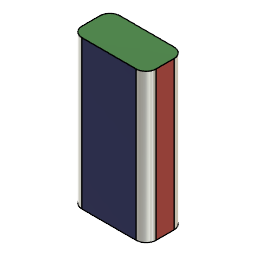
Raven Electronics Assembly (Autodesk Fusion 360 archive; units mm, degrees)
design "2s3000Mah Copy"
Autodesk Fusion 360 part; units mm, degrees
sketch "Sketch1" plane through (0, 0, 0) normal (0, 0, 1) x (1, 0, 0)
  line L0 (18.5, 9.5) -> (-18.5, 9.5)
  line L1 (-18.5, 9.5) -> (-18.5, -9.5)
  line L2 (-18.5, -9.5) -> (18.5, -9.5)
  line L3 (18.5, -9.5) -> (18.5, 9.5)
  line L4 (18.5, 9.5) -> (-18.5, -9.5) construction
  line L5 (-18.5, 9.5) -> (18.5, -9.5) construction
  dimension "d3" = 19
  dimension "d4" = 37
  constraint horizontal L0
  constraint perpendicular L0 L1
  constraint parallel L0 L2
  constraint parallel L1 L3
  constraint coincident L4 origin
  constraint coincident L5 origin
  measures "d3" distance of L0.end L1.end
  measures "d4" distance of L0.start L0.end
extrude "Extrude1" add sketch "Sketch1" along normal blind 74
fillet "Fillet1" radius 5 4 edges at (-18.5, -9.5, 37) (18.5, 9.5, 37) (18.5, -9.5, 37) (-18.5, 9.5, 37)

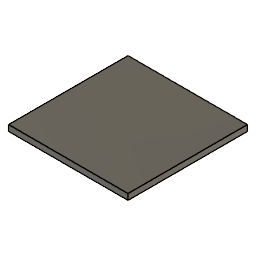
design "Electronics Case Top"
Autodesk Fusion 360 part; units mm, degrees
sketch "Sketch1" plane through (0, 0, 0) normal (0, 0, 1) x (1, 0, 0)
  line L0 (0, 0) -> (60, 0)
  line L1 (60, 0) -> (60, 60)
  line L2 (60, 60) -> (0, 60)
  line L3 (0, 60) -> (0, 0)
  dimension "d1" = 60
  dimension "d2" = 60
  constraint horizontal L0
  constraint vertical L1
  constraint horizontal L2
  constraint vertical L3
  constraint coincident L0.start L3.end
  measures "d1" distance of L0.start L0.end
  measures "d2" distance of L0.start L2.end
extrude "Extrude1" add sketch "Sketch1" along normal blind 3

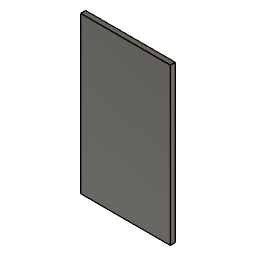
design "Electronics Case Right Wall"
Autodesk Fusion 360 part; units mm, degrees
sketch "Sketch1" plane through (0, 0, 0) normal (0, 1, 0) x (1, 0, 0)
  line L0 (0, 0) -> (54, 0)
  line L1 (54, 0) -> (54, -94)
  line L2 (54, -94) -> (0, -94)
  line L3 (0, -94) -> (0, 0)
  dimension "d1" = 54
  dimension "d2" = 94
  constraint horizontal L0
  constraint vertical L1
  constraint horizontal L2
  constraint vertical L3
  constraint coincident L0.start L3.end
  measures "d1" distance of L0.start L0.end
  measures "d2" distance of L0.start L2.end
extrude "Extrude1" add sketch "Sketch1" along normal blind 3

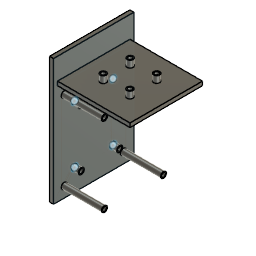
design "Electronics Case Back wall"
Autodesk Fusion 360 part; units mm, degrees
sketch "Sketch1" plane through (0, 0, 0) normal (1, 0, 0) x (0, 1, 0)
  line L0 (0, 0) -> (60, 0)
  line L1 (60, 0) -> (60, 94)
  line L2 (60, 94) -> (0, 94)
  line L3 (0, 94) -> (0, 0)
  dimension "d1" = 60
  dimension "d2" = 94
  constraint horizontal L0
  constraint vertical L1
  constraint horizontal L2
  constraint vertical L3
  constraint coincident L0.start L3.end
  measures "d1" distance of L0.start L0.end
  measures "d2" distance of L0.start L2.end
extrude "Extrude1" add sketch "Sketch1" along normal blind 3
sketch "Sketch2" plane through (3, 0, 0) normal (1, 0, 0) x (0, 1, 0)
  line L0 (0, 94) -> (0, 0)
  line L1 (0, 0) -> (60, 0)
  line L2 (60, 0) -> (60, 94)
  line L3 (60, 94) -> (0, 94)
  line L4 (0, 0) -> (0, 75)
  line L5 (0, 75) -> (60, 75)
  line L6 (60, 75) -> (60, 78)
  line L7 (60, 78) -> (0, 78)
  line L8 (0, 78) -> (0, 75)
  dimension "d5" = 75
  dimension "d6" = 60
  dimension "d7" = 3
  constraint coincident L0.end L1.start
  constraint perpendicular L1 L4
  constraint horizontal L5
  constraint vertical L6
  constraint horizontal L7
  constraint vertical L8
  measures "d5" distance of L0.end L4.end
  measures "d6" distance of L4.end L5.end
  measures "d7" distance of L4.end L7.end
extrude "Extrude2" add sketch "Sketch2" along normal blind 54 contours L0 L2 L5 L6 L7 L8
sketch "Sketch3" plane through (0, 0, 0) normal (0, -1, 0) x (1, 0, 0)
  line L0 (0, 94) -> (0, 0)
  line L1 (0, 0) -> (3, 0)
  line L2 (3, 0) -> (3, 75)
  line L3 (3, 75) -> (57, 75)
  line L4 (57, 75) -> (57, 78)
  line L5 (57, 78) -> (3, 78)
  line L6 (3, 78) -> (3, 94)
  line L7 (3, 94) -> (0, 94)
  line L8 (3, 75) -> (57, 75)
  line L9 (57, 75) -> (57, 78)
  line L10 (57, 78) -> (3, 78)
  line L11 (3, 78) -> (3, 75)
  constraint horizontal L8
  constraint vertical L9
  constraint horizontal L10
  constraint vertical L11
  constraint coincident L4.end L5.start
  constraint coincident L2.end L3.start
extrude "Extrude3" cut sketch "Sketch3" against normal blind 3 contours L3 L4 L5 L8 L9 L10 L11
sketch "Sketch4" plane through (0, 60, 0) normal (0, 1, 0) x (-1, 0, 0)
  line L0 (0, 0) -> (0, 94)
  line L1 (0, 94) -> (-3, 94)
  line L2 (-3, 94) -> (-3, 78)
  line L3 (-3, 78) -> (-57, 78)
  line L4 (-57, 78) -> (-57, 75)
  line L5 (-57, 75) -> (-3, 75)
  line L6 (-3, 75) -> (-3, 0)
  line L7 (-3, 0) -> (0, 0)
  line L8 (-57, 75) -> (-3, 75)
  line L9 (-3, 75) -> (-3, 78)
  line L10 (-3, 78) -> (-57, 78)
  line L11 (-57, 78) -> (-57, 75)
  constraint horizontal L8
  constraint vertical L9
  constraint horizontal L10
  constraint vertical L11
  constraint coincident L2.end L3.start
  constraint coincident L4.end L5.start
extrude "Extrude4" cut sketch "Sketch4" against normal blind 3 contours L3 L4 L5 L8 L9 L10 L11
sketch "Sketch5" plane through (3, 0, 0) normal (1, 0, 0) x (0, 1, 0)
  line L0 (57, 75) -> (3, 75)
  line L1 (3, 75) -> (3, 78)
  line L2 (3, 78) -> (57, 78)
  line L3 (57, 78) -> (57, 75)
  line L4 (60, 0) -> (60, 94)
  line L5 (60, 94) -> (0, 94)
  line L6 (0, 94) -> (0, 0)
  line L7 (0, 0) -> (60, 0)
sketch "Sketch6" plane through (3, 0, 0) normal (1, 0, 0) x (0, 1, 0)
  circle A0 centre (44.31, 16.105) radius 1.5
  circle A1 centre (44.31, 16.105) radius 2.25
  circle A2 centre (15.69, 16.105) radius 1.5
  circle A3 centre (15.69, 16.105) radius 2.25
  circle A4 centre (15.69, 58.895) radius 1.5
  circle A5 centre (15.69, 58.895) radius 2.25
  circle A6 centre (44.31, 58.895) radius 1.5
  circle A7 centre (44.31, 58.895) radius 2.25
  dimension "d25" = 3
  dimension "d26" = 4.5
  dimension "d27" = 28.62
  dimension "d28" = 3
  dimension "d29" = 4.5
  dimension "d30" = 42.79
  dimension "d31" = 3
  dimension "d32" = 4.5
  dimension "d33" = 42.79
  dimension "d34" = 3
  dimension "d35" = 4.5
  constraint concentric A0 A1
  constraint concentric A2 A3
  constraint concentric A4 A5
  constraint concentric A6 A7
  measures "d25" diameter of A0
  measures "d26" diameter of A1
  measures "d27" distance of A0.centre A2.centre
  measures "d28" diameter of A2
  measures "d29" diameter of A3
  measures "d30" distance of A2.centre A4.centre
  measures "d31" diameter of A4
  measures "d32" diameter of A5
  measures "d33" distance of A0.centre A6.centre
  measures "d34" diameter of A6
  measures "d35" diameter of A7
extrude "Extrude6" add sketch "Sketch6" along normal blind 5
sketch "Sketch7" plane through (0, 0, 78) normal (0, 0, 1) x (-1, 0, 0)
  line L0 (-57, -57) -> (-3, -57)
  line L1 (-3, -57) -> (-3, -3)
  line L2 (-3, -3) -> (-57, -3)
  line L3 (-57, -3) -> (-57, -57)
  line L4 (-57, -3) -> (-57, -20)
  line L5 (-57, -20) -> (-39.9, -20)
  circle A0 centre (-39.9, -20) radius 1.5
  circle A1 centre (-39.9, -20) radius 2.25
  line L6 (-39.9, -20) -> (-20.1, -20)
  circle A2 centre (-20.1, -20) radius 1.5
  circle A3 centre (-20.1, -20) radius 2.25
  line L7 (-20.1, -20) -> (-20.1, -40)
  circle A4 centre (-20.1, -40) radius 1.5
  circle A5 centre (-20.1, -40) radius 2.25
  line L8 (-39.9, -20) -> (-39.9, -40)
  circle A6 centre (-39.9, -40) radius 1.5
  circle A7 centre (-39.9, -40) radius 2.25
  dimension "d38" = 17
  dimension "d39" = 17.1
  dimension "d40" = 3
  dimension "d41" = 4.5
  dimension "d42" = 19.8
  dimension "d43" = 3
  dimension "d44" = 4.5
  dimension "d45" = 20
  dimension "d46" = 3
  dimension "d47" = 4.5
  dimension "d48" = 20
  dimension "d49" = 3
  dimension "d50" = 4.5
  constraint coincident L2.end L3.start
  constraint perpendicular L2 L4
  constraint perpendicular L4 L5
  constraint coincident L5.end A0.centre
  constraint concentric A0 A1
  constraint parallel L5 L6
  constraint coincident L6.end A2.centre
  constraint concentric A2 A3
  constraint perpendicular L6 L7
  constraint coincident L7.end A4.centre
  constraint concentric A4 A5
  constraint perpendicular L6 L8
  constraint coincident L8.end A6.centre
  constraint concentric A6 A7
  measures "d38" distance of L2.end L4.end
  measures "d39" distance of L4.end L5.end
  measures "d40" diameter of A0
  measures "d41" diameter of A1
  measures "d42" distance of L5.end L6.end
  measures "d43" diameter of A2
  measures "d44" diameter of A3
  measures "d45" distance of L6.end L7.end
  measures "d46" diameter of A4
  measures "d47" diameter of A5
  measures "d48" distance of L5.end L8.end
  measures "d49" diameter of A6
  measures "d50" diameter of A7
extrude "Extrude7" add sketch "Sketch7" along normal blind 5 contours L5 A0 A1 L6 | L5 A0 A1 L8 | A0 A1 L6 L8 | L6 A2 A3 L7 | L6 A2 A3 L7 | A5 | A7
sketch "Sketch8" plane through (3, 0, 0) normal (1, 0, 0) x (0, 1, 0)
  line L0 (0, 0) -> (8, 0)
  line L1 (8, 0) -> (8, 8)
  circle A0 centre (8, 8) radius 1.5
  circle A1 centre (8, 8) radius 2.25
  line L2 (60, 0) -> (52, 0)
  line L3 (52, 0) -> (52, 8)
  line L4 (52, 8) -> (60, 8)
  line L5 (60, 8) -> (60, 0)
  circle A2 centre (52, 8) radius 1.5
  circle A3 centre (52, 8) radius 2.25
  line L6 (60, 75) -> (52, 75)
  line L7 (52, 75) -> (52, 67)
  line L8 (52, 67) -> (60, 67)
  line L9 (60, 67) -> (60, 75)
  circle A4 centre (52, 67) radius 1.5
  circle A5 centre (52, 67) radius 2.25
  line L10 (0, 75) -> (8, 75)
  line L11 (8, 75) -> (8, 67)
  line L12 (8, 67) -> (0, 67)
  line L13 (0, 67) -> (0, 75)
  circle A6 centre (8, 67) radius 1.5
  circle A7 centre (8, 67) radius 2.25
  dimension "d53" = 8
  dimension "d54" = 8
  dimension "d55" = 3
  dimension "d56" = 4.5
  dimension "d57" = 8
  dimension "d58" = 8
  dimension "d59" = 3
  dimension "d60" = 4.5
  dimension "d61" = 8
  dimension "d62" = 8
  dimension "d63" = 3
  dimension "d64" = 4.5
  dimension "d65" = 8
  dimension "d66" = 8
  dimension "d67" = 3
  dimension "d68" = 4.5
  constraint coincident L0.start origin
  constraint horizontal L0
  constraint perpendicular L0 L1
  constraint coincident L1.end A0.centre
  constraint concentric A0 A1
  constraint horizontal L2
  constraint vertical L3
  constraint horizontal L4
  constraint vertical L5
  constraint coincident L3.end L4.start
  constraint concentric A2 A3
  constraint horizontal L6
  constraint vertical L7
  constraint horizontal L8
  constraint vertical L9
  constraint coincident L7.end L8.start
  constraint concentric A4 A5
  constraint horizontal L10
  constraint vertical L11
  constraint horizontal L12
  constraint vertical L13
  constraint coincident L11.end L12.start
  constraint concentric A6 A7
  measures "d53" distance of L0.start L0.end
  measures "d54" distance of L0.end L1.end
  measures "d55" diameter of A0
  measures "d56" diameter of A1
  measures "d57" distance of L2.start L2.end
  measures "d58" distance of L2.start L4.end
  measures "d59" diameter of A2
  measures "d60" diameter of A3
  measures "d61" distance of L6.start L6.end
  measures "d62" distance of L6.start L8.end
  measures "d63" diameter of A4
  measures "d64" diameter of A5
  measures "d65" distance of L10.start L10.end
  measures "d66" distance of L10.start L12.end
  measures "d67" diameter of A6
  measures "d68" diameter of A7
extrude "Extrude8" add sketch "Sketch8" along normal blind 30 contours A1 | L3 L4 A2 A3 | L3 L4 A2 A3 | L7 L8 A4 A5 | L7 L8 A4 A5 | L11 L12 A6 A7 | L11 L12 A6 A7

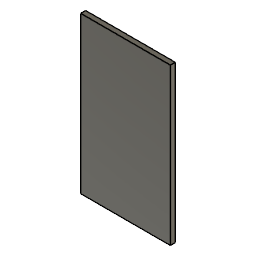
design "Electronics Case Left wall"
Autodesk Fusion 360 part; units mm, degrees
sketch "Sketch1" plane through (0, 0, 0) normal (0, 1, 0) x (1, 0, 0)
  line L0 (0, 0) -> (54, 0)
  line L1 (54, 0) -> (54, -94)
  line L2 (54, -94) -> (0, -94)
  line L3 (0, -94) -> (0, 0)
  dimension "d1" = 54
  dimension "d2" = 94
  constraint horizontal L0
  constraint vertical L1
  constraint horizontal L2
  constraint vertical L3
  constraint coincident L0.start L3.end
  measures "d1" distance of L0.start L0.end
  measures "d2" distance of L0.start L2.end
extrude "Extrude1" add sketch "Sketch1" along normal blind 3

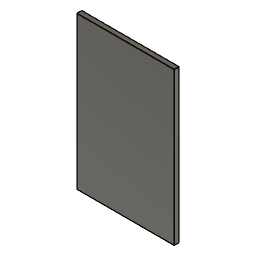
design "Electronics Case Front Wall"
Autodesk Fusion 360 part; units mm, degrees
sketch "Sketch1" plane through (0, 0, 0) normal (0, 1, 0) x (1, 0, 0)
  line L0 (0, 0) -> (60, 0)
  line L1 (60, 0) -> (60, -94)
  line L2 (60, -94) -> (0, -94)
  line L3 (0, -94) -> (0, 0)
  dimension "d1" = 60
  dimension "d2" = 94
  constraint horizontal L0
  constraint vertical L1
  constraint horizontal L2
  constraint vertical L3
  constraint coincident L0.start L3.end
  measures "d1" distance of L0.start L0.end
  measures "d2" distance of L0.start L2.end
extrude "Extrude1" add sketch "Sketch1" along normal blind 3

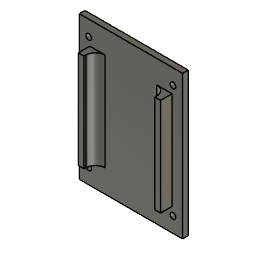
design "Electronics case internal battery shelf"
Autodesk Fusion 360 part; units mm, degrees
sketch "Sketch1" plane through (0, 0, 0) normal (0, 1, 0) x (1, 0, 0)
  line L0 (0, 0) -> (54, 0)
  line L1 (54, 0) -> (54, -75)
  line L2 (54, -75) -> (0, -75)
  line L3 (0, -75) -> (0, 0)
  dimension "d1" = 54
  dimension "d2" = 75
  constraint horizontal L0
  constraint vertical L1
  constraint horizontal L2
  constraint vertical L3
  constraint coincident L0.start L3.end
  measures "d1" distance of L0.start L0.end
  measures "d2" distance of L0.start L2.end
extrude "Extrude1" add sketch "Sketch1" along normal blind 3
sketch "Sketch2" plane through (0, 0, 0) normal (0, -1, 0) x (1, 0, 0)
  line L0 (54, 75) -> (0, 75)
  line L1 (0, 75) -> (0, 0)
  line L2 (0, 0) -> (54, 0)
  line L3 (54, 0) -> (54, 75)
  line L4 (54, 75) -> (49, 75)
  line L5 (54, 67) -> (54, 75)
  circle A0 centre (49, 67) radius 1.5
  line L6 (0, 75) -> (5, 75)
  line L7 (0, 67) -> (0, 75)
  circle A1 centre (5, 67) radius 1.5
  line L8 (0, 0) -> (5, 0)
  line L9 (0, 8) -> (0, 0)
  circle A2 centre (5, 8) radius 1.5
  line L10 (54, 0) -> (49, 0)
  line L11 (54, 8) -> (54, 0)
  circle A3 centre (49, 8) radius 1.5
  dimension "d5" = 5
  dimension "d6" = 8
  dimension "d7" = 3
  dimension "d8" = 5
  dimension "d9" = 8
  dimension "d10" = 3
  dimension "d11" = 5
  dimension "d12" = 8
  dimension "d13" = 3
  dimension "d14" = 5
  dimension "d15" = 8
  dimension "d16" = 3
  constraint horizontal L4
  constraint vertical L5
  constraint coincident L0.start L3.end
  constraint horizontal L6
  constraint vertical L7
  constraint coincident L0.end L1.start
  constraint horizontal L8
  constraint vertical L9
  constraint coincident L1.end L2.start
  constraint horizontal L10
  constraint vertical L11
  constraint coincident L2.end L3.start
  measures "d5" distance of L0.start L4.end
  measures "d6" distance of L0.start L5.start
  measures "d7" diameter of A0
  measures "d8" distance of L0.end L6.end
  measures "d9" distance of L0.end L7.start
  measures "d10" diameter of A1
  measures "d11" distance of L1.end L8.end
  measures "d12" distance of L1.end L9.start
  measures "d13" diameter of A2
  measures "d14" distance of L2.end L10.end
  measures "d15" distance of L2.end L11.start
  measures "d16" diameter of A3
extrude "Extrude2" cut sketch "Sketch2" against normal blind 50 contours A0 | A1 | A2 | A3
sketch "Sketch3" plane through (0, 0, 0) normal (0, -1, 0) x (1, 0, 0)
  circle A0 centre (49, 8) radius 1.5
  circle A1 centre (49, 67) radius 1.5
  circle A2 centre (5, 8) radius 1.5
  circle A3 centre (5, 67) radius 1.5
  line L0 (54, 75) -> (0, 75)
  line L1 (0, 75) -> (0, 0)
  line L2 (0, 0) -> (54, 0)
  line L3 (54, 0) -> (54, 75)
  line L4 (0, 75) -> (8.5, 75)
  line L5 (0, 0) -> (8.5, 0)
  line L6 (8.5, 12) -> (5.5, 12)
  line L7 (5.5, 12) -> (5.5, 63)
  line L8 (5.5, 63) -> (8.5, 63)
  line L9 (8.5, 63) -> (8.5, 12)
  line L10 (54, 75) -> (45.5, 75)
  line L11 (54, 0) -> (45.5, 0)
  line L12 (45.5, 12) -> (48.5, 12)
  line L13 (48.5, 12) -> (48.5, 63)
  line L14 (48.5, 63) -> (45.5, 63)
  line L15 (45.5, 63) -> (45.5, 12)
  dimension "d19" = 8.5
  dimension "d20" = 8.5
  dimension "d21" = 12
  dimension "d22" = 3
  dimension "d23" = 51
  dimension "d24" = 8.5
  dimension "d26" = 8.5
  dimension "d27" = 12
  dimension "d28" = 3
  dimension "d29" = 51
  constraint coincident L0.end L1.start
  constraint perpendicular L1 L4
  constraint coincident L1.end L2.start
  constraint perpendicular L1 L5
  constraint horizontal L6
  constraint vertical L7
  constraint horizontal L8
  constraint vertical L9
  constraint coincident L0.start L3.end
  constraint perpendicular L3 L10
  constraint coincident L2.end L3.start
  constraint perpendicular L3 L11
  constraint horizontal L12
  constraint vertical L13
  constraint horizontal L14
  constraint vertical L15
  measures "d19" distance of L0.end L4.end
  measures "d20" distance of L1.end L5.end
  measures "d21" distance of L5.end L6.start
  measures "d22" distance of L6.start L6.end
  measures "d23" distance of L6.start L8.end
  measures "d24" distance of L0.start L10.end
  measures "d26" distance of L2.end L11.end
  measures "d27" distance of L11.end L12.start
  measures "d28" distance of L12.start L12.end
  measures "d29" distance of L12.start L14.end
extrude "Extrude3" add sketch "Sketch3" along normal blind 6 contours L6 L7 L8 L9 | L12 L13 L14 L15
fillet "Fillet1" radius 5 2 edges at (8.5, 0, 37.5) (45.5, 0, 37.5)

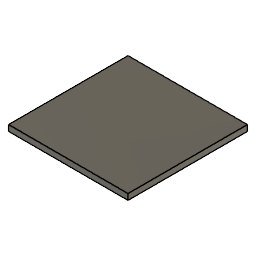
design "Electonics Case Base"
Autodesk Fusion 360 part; units mm, degrees
sketch "Sketch1" plane through (0, 0, 0) normal (0, 0, 1) x (1, 0, 0)
  line L0 (0, 0) -> (60, 0)
  line L1 (60, 0) -> (60, 60)
  line L2 (60, 60) -> (0, 60)
  line L3 (0, 60) -> (0, 0)
  dimension "d1" = 60
  dimension "d2" = 60
  constraint horizontal L0
  constraint vertical L1
  constraint horizontal L2
  constraint vertical L3
  constraint coincident L0.start L3.end
  measures "d1" distance of L0.start L0.end
  measures "d2" distance of L0.start L2.end
extrude "Extrude1" add sketch "Sketch1" along normal blind 3
